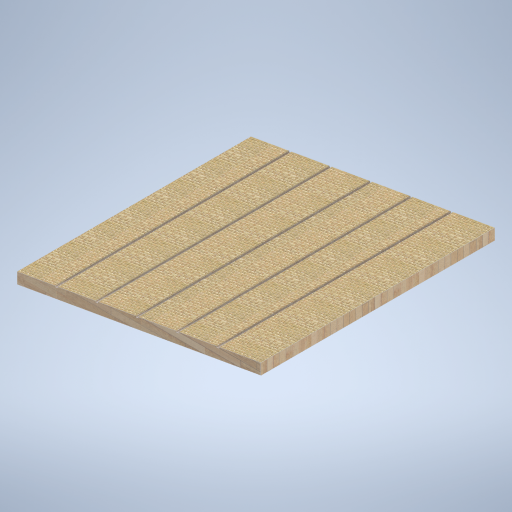
# Autodesk Inventor part: eave_panel_side
Saved by Autodesk Inventor 2024.2 (Build 282272000, 272)
## iProperties
Created: 2024-05-24
Part Number: eave_panel_side
Material: Wood (Maple)
Document SubType Name: Modeling
Designer: LOSTER_1
Density: 0.67 g/cm^3
Appearance: Natural Maple - Glossy Dark Tint
Author: LOSTER_1
Autodesk Inventor part; units mm, degrees
ref_plane "YZ Plane" through (0, 0, 0) normal (1, 0, 0) x (0, 1, 0)
ref_plane "XZ Plane" through (0, 0, 0) normal (0, 1, 0) x (-1, 0, 0)
ref_plane "XY Plane" through (0, 0, 0) normal (0, 0, 1) x (1, 0, 0)
sketch "Sketch1" plane through (0, 0, 0) normal (1, 0, 0) x (0, 1, 0)
  line L0 (-50, 1055) -> (50, 1055)
  line L1 (50, 1055) -> (50, -1055)
  line L2 (50, -1055) -> (-50, -1055)
  line L3 (-50, -1055) -> (-50, 1055)
  line L4 (-50, 1055) -> (50, -1055) construction
  line L5 (50, 1055) -> (-50, -1055) construction
  point P0 (0, 0)
  dimension "d0" = 100
  dimension "d1" = 2110
  constraints: 12 end point, 2 midpoint, 2 parallel, 1 horizontal, 1 perpendicular
  measures "d0" distance of L1.end L2.end
  measures "d1" distance of L0.end L1.end
ref_plane "Work Plane2" through (-2200, 50, 1055) normal (-1, 0, 0) x (0, 0, -1)
ref_plane "Work Plane1" through (0, 50, 1055) normal (-1, 0, 0) x (0, 0, -1)
sketch "Sketch2" plane through (-2200, 50, 1055) normal (-1, 0, 0) x (0, 0, -1)
  line L0 (2110, 0) -> (2110, 100) projected
  point P0 (1055, 50)
ref_plane "Work Plane3" through (-2200, 50, -1055) normal (0, 0, 1) x (0, -1, 0)
sketch "Sketch3" plane through (-2200, 50, -1055) normal (0, 0, 1) x (0, -1, 0)
  line L0 (0, 2200) -> (100, 2200) projected
  line L1 (0, 0) -> (100, 0) projected
  line L2 (0, 2200) -> (387.9194, 0)
  line L3 (0, 2200) -> (2233.9385, 2200) construction
  line L4 (100, 2200) -> (487.9194, 0)
  line L5 (100, 2200) -> (2333.9385, 2200) construction
  line L6 (487.9194, 0) -> (387.9194, 0)
  point P0 (50, 2200)
  dimension "d3" = 80
  dimension "d4" = 80
  constraints: 10 end point, 3 horizontal, 2 equal length
  measures "d3" angle of L2 L3
  measures "d4" angle of L4 L5
extrude "Extrusion1" add sketch "Sketch3" along normal blind 2110
sketch "Sketch4" plane through (-2200, 50, 1055) normal (0, 0, 1) x (1, 0, 0)
  line L0 (0, -387.9194) -> (0, -487.9194) projected
  line L1 (0, -387.9194) -> (344.6827, -327.1425)
  line L2 (2200, 0) -> (0, -387.9194) projected
  line L3 (344.6827, -327.1425) -> (344.6827, -337.3172)
  line L4 (344.6827, -337.3172) -> (364.7974, -333.7704)
  line L5 (364.7974, -333.7704) -> (364.7974, -323.5957)
  line L6 (364.7974, -323.5957) -> (709.4801, -262.8189)
  line L7 (709.4801, -262.8189) -> (709.4801, -272.9936)
  line L8 (709.4801, -272.9936) -> (728.9354, -269.5631)
  line L9 (728.9354, -269.5631) -> (728.9354, -259.3884)
  line L10 (728.9354, -259.3884) -> (1073.6181, -198.6115)
  line L11 (1073.6181, -198.6115) -> (1073.6181, -208.7862)
  line L12 (1073.6181, -208.7862) -> (1092.9901, -205.3704)
  line L13 (1092.9901, -205.3704) -> (1092.9901, -195.1957)
  line L14 (1092.9901, -195.1957) -> (1437.6728, -134.4189)
  line L15 (1437.6728, -134.4189) -> (1437.6728, -144.5935)
  line L16 (1437.6728, -144.5935) -> (1456.9375, -141.1967)
  line L17 (1456.9375, -141.1967) -> (1456.9375, -131.022)
  line L18 (1456.9375, -131.022) -> (1801.6202, -70.2451)
  line L19 (1801.6202, -70.2451) -> (1801.6202, -80.4198)
  line L20 (1801.6202, -80.4198) -> (1821.3275, -76.9449)
  line L21 (1821.3275, -76.9449) -> (1821.3275, -66.7702)
  line L22 (1821.3275, -66.7702) -> (2200, 0)
  line L23 (1821.3275, -66.7702) -> (344.6827, -327.1425)
  point P0 (2200, -50)
  dimension "d7" = 350
  dimension "d8" = 350
  dimension "d9" = 350
  dimension "d10" = 350
  dimension "d11" = 350
  constraints: 44 end point, 18 point on line, 10 parallel, 2 collinear, 1 vertical
  measures "d7" distance of L0.start L1.end
  measures "d8" distance of L5.end L6.end
  measures "d9" distance of L9.end L10.end
  measures "d10" distance of L13.end L14.end
  measures "d11" distance of L17.end L18.end
extrude "Extrusion2" cut sketch "Sketch4" against normal through all
body "Solid1"
